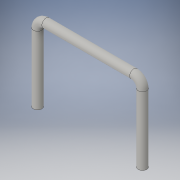
# Autodesk Inventor part: Large_Staple
Saved by Autodesk Inventor 2016 (Build 200138000, 138)
## iProperties
Created: 2017-11-09
Part Number: Large_Staple
Material: Generic
Document SubType Name: Modeling
Designer: shen95841
Density: 1 g/cm^3
Appearance: Default
Author: shen95841
Autodesk Inventor part; units mm, degrees
ref_plane "YZ Plane" through (0, 0, 0) normal (1, 0, 0) x (0, 1, 0)
ref_plane "XZ Plane" through (0, 0, 0) normal (0, 1, 0) x (-1, 0, 0)
ref_plane "XY Plane" through (0, 0, 0) normal (0, 0, 1) x (1, 0, 0)
sketch "Sketch1" plane through (0, 0, 0) normal (0, 0, 1) x (1, 0, 0)
  line L0 (0, 0) -> (0, 11.1252)
  line L1 (1.397, 12.5222) -> (15.748, 12.5222)
  line L2 (17.145, 11.1252) -> (17.145, 0)
  arc A0 (1.397, 12.5222) -> (0, 11.1252) centre (1.397, 11.1252) ccw
  arc A1 (17.145, 11.1252) -> (15.748, 12.5222) centre (15.748, 11.1252) ccw
  point P0 (0, 12.5222)
  point P1 (17.145, 12.5222)
  dimension "d0" = 12.5222
  dimension "d1" = 17.145
  dimension "d2" = 1.397
  constraints: 6 end point, 4 point on circle, 4 point on line, 4 tangent, 2 centre point, 2 perpendicular, 1 equal radius, 1 vertical
  measures "d0" distance of L0.start point (0, 12.522)
  measures "d1" distance of point (0, 12.522) point (17.145, 12.522)
  measures "d2" radius of A0
sketch "Sketch2" plane through (0, 0, 0) normal (0, 1, 0) x (-1, 0, 0)
  circle A0 centre (0, 0) radius 0.6985
  dimension "d3" = 1.397
  constraints: 1 centre point, 1 coincident
  measures "d3" diameter of A0
sweep "Sweep1" add profiles "Sketch2" path "Sketch1" path curves L0 A0 L1 A1 L2
body "Solid1"
